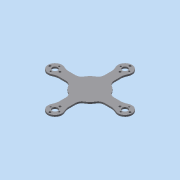
# Autodesk Inventor part: outline
Saved by Autodesk Inventor 2015 (Build 190159000, 159)
## iProperties
Created: 2016-01-29
Part Number: outline
Material: Generic
Document SubType Name: Modeling
Designer: Raphael
Density: 1 g/cm^3
Appearance: Default
Author: Raphael
Autodesk Inventor part; units mm, degrees
ref_plane "YZ Plane" through (0, 0, 0) normal (1, 0, 0) x (0, 1, 0)
ref_plane "XZ Plane" through (0, 0, 0) normal (0, 1, 0) x (-1, 0, 0)
ref_plane "XY Plane" through (0, 0, 0) normal (0, 0, 1) x (1, 0, 0)
sketch "Sketch1" plane through (0, 0, 0) normal (0, 1, 0) x (-1, 0, 0)
  line L0 (15.1438, 4.7625) -> (29.7948, 4.7625)
  line L1 (29.7948, -4.7625) -> (15.1438, -4.7625)
  line L2 (77.295, 0) -> (-61.795, 0) projected
  line L3 (0, -61.795) -> (0, 77.295) projected
  line L4 (-4.7625, 15.1438) -> (-4.7625, 29.7948)
  line L5 (4.7625, 29.7948) -> (4.7625, 15.1438)
  line L6 (-15.1438, -4.7625) -> (-29.7948, -4.7625)
  line L7 (-29.7948, 4.7625) -> (-15.1438, 4.7625)
  line L8 (4.7625, -15.1438) -> (4.7625, -29.7948)
  line L9 (-4.7625, -29.7948) -> (-4.7625, -15.1438)
  arc A0 (-4.7625, 15.1438) -> (-15.1438, 4.7625) centre (0, 0) ccw
  arc A1 (-15.1438, -4.7625) -> (-4.7625, -15.1438) centre (0, 0) ccw
  arc A2 (4.7625, -15.1438) -> (15.1438, -4.7625) centre (0, 0) ccw
  arc A3 (15.1438, 4.7625) -> (4.7625, 15.1438) centre (0, 0) ccw
  arc A4 (-29.7948, 4.7625) -> (-29.7948, -4.7625) centre (-34.925, 0) ccw
  arc A5 (4.7625, 29.7948) -> (-4.7625, 29.7948) centre (0, 34.925) ccw
  arc A6 (29.7948, -4.7625) -> (29.7948, 4.7625) centre (34.925, 0) ccw
  arc A7 (-4.7625, -29.7948) -> (4.7625, -29.7948) centre (0, -34.925) ccw
  dimension "d9" = 9.525
  dimension "d12" = 360
  dimension "d14" = 15.875
  dimension "d17" = 34.925
  dimension "d18" = 34.925
  dimension "d19" = 34.925
  dimension "d20" = 34.925
  dimension "d21" = 14
  constraints: 16 end point, 16 point on circle, 8 centre point, 3 point on line, 1 coincident, 1 horizontal, 1 parallel, 26 other
  measures "d9" distance between parallel lines of L0 L1
  measures "d14" radius of A1
  measures "d17" distance of point (0, 0) A6.centre
  measures "d18" distance of A7.centre point (0, 0)
  measures "d19" distance of A4.centre point (0, 0)
  measures "d20" distance of point (0, 0) A5.centre
  measures "d21" diameter of A5
extrude "Extrusion1" add sketch "Sketch1" along normal blind 1.6
fillet "Fillet1" radius 6.35 8 edges at (4.7625, 0.8, 15.1438) (15.1438, 0.8, 4.7625) (15.1438, 0.8, -4.7625) (4.7625, 0.8, -15.1438) (-4.7625, 0.8, -15.1438) (-15.1438, 0.8, -4.7625) (-15.1438, 0.8, 4.7625) (-4.7625, 0.8, 15.1438)
fillet "Fillet1" radius 12.7 8 edges at (29.7948, 0.8, 4.7625) (29.7948, 0.8, -4.7625) (4.7625, 0.8, -29.7948) (-4.7625, 0.8, -29.7948) (-29.7948, 0.8, -4.7625) (-29.7948, 0.8, 4.7625) (-4.7625, 0.8, 29.7948) (4.7625, 0.8, 29.7948)
sketch "Sketch2" plane through (0, 1.6, 0) normal (0, 1, 0) x (1, 0, 0)
  arc A0 (6.2049, 31.6848) -> (-6.2049, 31.6848) centre (0, 34.925) ccw projected
  circle A1 centre (-3.7123, 38.6373) radius 1.1
  circle A2 centre (3.7123, 38.6373) radius 1.1
  circle A3 centre (3.7123, 31.2127) radius 1.1
  circle A4 centre (-3.7123, 31.2127) radius 1.1
  line L0 (3.7123, 38.6373) -> (-3.7123, 31.2127)
  line L1 (3.7123, 31.2127) -> (-3.7123, 38.6373)
  circle A5 centre (0, 34.925) radius 2.54
  circle A6 centre (3.0052, 31.9198) radius 1.1
  circle A7 centre (-3.0052, 37.9302) radius 1.1
  circle A8 centre (3.0052, 37.9302) radius 1.1
  circle A9 centre (-3.0052, 31.9198) radius 1.1
  line L2 (3.0052, 37.9302) -> (-3.0052, 31.9198)
  line L3 (-3.0052, 37.9302) -> (3.0052, 31.9198)
  line L4 (-4.4901, 37.8595) -> (-3.783, 37.1524)
  line L5 (-2.8284, 39.2921) -> (-2.2387, 38.7192)
  line L6 (2.2274, 38.708) -> (2.9345, 39.4151)
  line L7 (3.783, 37.1524) -> (4.4901, 37.8595)
  line L8 (3.783, 32.6976) -> (4.4901, 31.9905)
  line L9 (2.9345, 30.4349) -> (2.2274, 31.142)
  line L10 (-2.9345, 30.4349) -> (-2.2274, 31.142)
  line L11 (-4.4901, 31.9905) -> (-3.783, 32.6976)
  point P0 (0, 0)
  dimension "d26" = 2.2
  dimension "d27" = 2.2
  dimension "d28" = 2.2
  dimension "d29" = 2.2
  dimension "d30" = 10.5
  dimension "d31" = 10.5
  dimension "d32" = 5.08
  dimension "d40" = 2.2
  dimension "d41" = 2.2
  dimension "d42" = 2.2
  dimension "d43" = 2.2
  dimension "d44" = 8.5
  dimension "d45" = 8.5
  constraints: 24 end point, 16 point on circle, 10 point on line, 9 centre point, 7 tangent, 6 midpoint, 1 coincident, 1 collinear, 1 horizontal alignment, 1 perpendicular
  measures "d26" diameter of A1
  measures "d27" diameter of A2
  measures "d28" diameter of A3
  measures "d29" diameter of A4
  measures "d30" distance of L1.start L1.end
  measures "d31" distance of L0.start L0.end
  measures "d32" diameter of A5
  measures "d40" diameter of A6
  measures "d41" diameter of A7
  measures "d42" diameter of A8
  measures "d43" diameter of A9
  measures "d44" distance of L2.start L2.end
  measures "d45" distance of L3.end L3.start
sketch "Sketch4" plane through (0, 1.6, 0) normal (0, 1, 0) x (1, 0, 0)
  arc A0 (6.2049, 31.6848) -> (-6.2049, 31.6848) centre (0, 34.925) ccw projected
  circle A1 centre (0, 34.925) radius 2.75
  circle A2 centre (0, 34.925) radius 5 construction
  circle A3 centre (0, 39.925) radius 1.1
  circle A4 centre (0, 29.925) radius 1.1
  line L0 (0, 58.695) -> (0, -58.695) projected
  circle A5 centre (0, 34.925) radius 4.25 construction
  circle A6 centre (-4.25, 34.925) radius 0.8
  circle A7 centre (4.25, 34.925) radius 0.8
  point P0 (0, 0)
  dimension "d46" = 5.5
  dimension "d47" = 10
  dimension "d48" = 2.2
  dimension "d49" = 2.2
  dimension "d50" = 8.5
  dimension "d51" = 1.6
  dimension "d52" = 1.6
  constraints: 7 centre point, 4 point on circle, 3 coincident, 2 horizontal alignment, 2 point on line
  measures "d46" diameter of A1
  measures "d47" diameter of A2
  measures "d48" diameter of A3
  measures "d49" diameter of A4
  measures "d50" diameter of A5
  measures "d51" diameter of A6
  measures "d52" diameter of A7
extrude "Extrusion3" cut sketch "Sketch4" against normal through all
pattern_circular "Circular Pattern2" count 4 over 360 about axis through (0, -10, 0) along (0, 1, 0) of "Extrusion3"
equation "\"d17\" = arm"
equation "\"d18\" = arm"
equation "\"d19\" = arm"
equation "\"d20\" = arm"
equation "\"arm\" = 34.925"
body "Solid1"
